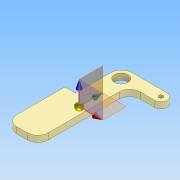
# Autodesk Inventor part: Selection_Lever 1
Saved by Autodesk Inventor 2018.1 (Build 221171000, 171)
## iProperties
Created: 2019-02-14
Part Number: Selection_Lever 1
Material: Nylon 6/6
Document SubType Name: Modeling
Designer: James
Density: 1.13 g/cm^3
Appearance: Nylon 6
Mass: 2.30209 g
Surface Area: 18.848 cm^2
Volume: 2.03725 cm^3
Author: James
Autodesk Inventor part; units mm, degrees
ref_plane "YZ Plane" through (0, 0, 0) normal (1, 0, 0) x (0, 1, 0)
ref_plane "XZ Plane" through (0, 0, 0) normal (0, 1, 0) x (-1, 0, 0)
ref_plane "XY Plane" through (0, 0, 0) normal (0, 0, 1) x (1, 0, 0)
sketch "Sketch1" plane through (0, 0, 0) normal (0, 0, 1) x (1, 0, 0)
  line L0 (0, 0) -> (10, 0)
  line L1 (10, 0) -> (10, 10)
  line L2 (10, 10) -> (0, 10)
  line L3 (0, 10) -> (0, 0)
  line L4 (10, 10) -> (25, 10)
  line L5 (25, 10) -> (25, 4)
  line L6 (25, 4) -> (10, 4)
  line L7 (10, 4) -> (10, 10)
  line L8 (10, 0) -> (0, 0)
  line L9 (0, 0) -> (0, -40)
  line L10 (0, -40) -> (10, -40)
  line L11 (10, -40) -> (10, 0)
  line L12 (0, -40) -> (-5, -40)
  line L13 (-5, -40) -> (-5, -12)
  line L14 (-5, -12) -> (0, -12)
  line L15 (0, -12) -> (0, -40)
  dimension "d0" = 10
  dimension "d2" = 15
  dimension "d3" = 6
  dimension "d5" = 28
  dimension "d6" = 5
  dimension "d7" = 10
  dimension "d30" = 22
  constraints: 32 end point, 8 parallel, 4 horizontal, 4 perpendicular, 1 coincident, 1 vertical alignment
  measures "d0" distance of L2.end L0.start
  measures "d2" distance of L1.end L4.end
  measures "d3" distance of L4.end L5.end
  measures "d5" distance of L12.end L13.end
  measures "d6" distance of L9.end L12.end
  measures "d7" distance of L9.end L10.end
  measures "d30" distance between parallel lines of L2 L14
extrude "Extrusion1" add sketch "Sketch1" along normal blind 3
fillet "Fillet1" radius 5 1 edges at (0, 10, 1.5)
fillet "Fillet2" radius 5 2 edges at (-5, -40, 1.5) (10, -40, 1.5)
fillet "Fillet3" radius 5 1 edges at (10, 4, 1.5)
full round fillet "Fillet4" first side at (18.3333, 4, 1) centre faces at (25, 6, 1) second side at (18.3333, 10, 1)
sketch "Sketch2" plane through (0, 0, 3) normal (0, 0, 1) x (1, 0, 0)
  arc A0 (22, 4) -> (22, 10) centre (22, 7) ccw projected
  point P0 (0, 0)
  constraints: 1 coincident
hole "Hole1" at (22, 7, 3) direction (0, 0, -1) diameter 2 end through all
sketch "Sketch3" plane through (0, 0, 3) normal (0, 0, 1) x (1, 0, 0)
  line L0 (22, 10) -> (5, 10) projected
  line L1 (0, 5) -> (0, -12) projected
  point P0 (0, 0)
  point P1 (5, 5)
  dimension "d20" = 5
  dimension "d31" = 5
  measures "d20" distance from line of point (5, 5) L0
  measures "d31" distance from line of point (5, 5) L1
hole "Hole2" at (5, 5, 3) direction (0, 0, -1) diameter 6.5 end through all
body "Solid1"
